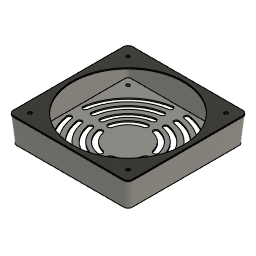
Fan Template - Tight Screen (Autodesk Fusion 360 design; units mm, degrees)
Autodesk Fusion 360 part; units mm, degrees
sketch "Base Master" plane through (0, 0, 0) normal (0, 0, 1) x (1, 0, 0)
  circle A0 centre (0, 0) radius 59.5
  line L0 (52.5, -52.5) -> (-52.5, -52.5) construction
  line L1 (-52.5, -52.5) -> (-52.5, 52.5) construction
  line L2 (-52.5, 52.5) -> (52.5, 52.5) construction
  line L3 (52.5, 52.5) -> (52.5, -52.5) construction
  line L4 (52.5, -52.5) -> (-52.5, 52.5) construction
  line L5 (-52.5, -52.5) -> (52.5, 52.5) construction
  circle A1 centre (-52.5, 52.5) radius 1.8
  circle A2 centre (52.5, 52.5) radius 1.8
  circle A3 centre (52.5, -52.5) radius 1.8
  circle A4 centre (-52.5, -52.5) radius 1.8
  line L6 (57.25, -60.25) -> (-57.25, -60.25)
  line L7 (-60.25, -57.25) -> (-60.25, 57.25)
  line L8 (-57.25, 60.25) -> (57.25, 60.25)
  line L9 (60.25, 57.25) -> (60.25, -57.25)
  line L10 (60.25, -60.25) -> (-60.25, 60.25) construction
  line L11 (-60.25, -60.25) -> (60.25, 60.25) construction
  arc A5 (-57.25, 60.25) -> (-60.25, 57.25) centre (-57.25, 57.25) ccw
  arc A6 (60.25, 57.25) -> (57.25, 60.25) centre (57.25, 57.25) ccw
  arc A7 (57.25, -60.25) -> (60.25, -57.25) centre (57.25, -57.25) ccw
  arc A8 (-60.25, -57.25) -> (-57.25, -60.25) centre (-57.25, -57.25) ccw
  line L12 (-61.85, -57.25) -> (-61.85, 57.25)
  arc A9 (-57.25, 61.85) -> (-61.85, 57.25) centre (-57.25, 57.25) ccw
  line L13 (-57.25, 61.85) -> (57.25, 61.85)
  arc A10 (61.85, 57.25) -> (57.25, 61.85) centre (57.25, 57.25) ccw
  line L14 (61.85, 57.25) -> (61.85, -57.25)
  arc A11 (57.25, -61.85) -> (61.85, -57.25) centre (57.25, -57.25) ccw
  line L15 (57.25, -61.85) -> (-57.25, -61.85)
  arc A12 (-61.85, -57.25) -> (-57.25, -61.85) centre (-57.25, -57.25) ccw
  dimension "d10" = 119
  dimension "d11" = 105
  dimension "d12" = 105
  dimension "d13" = 3.6
  dimension "d14" = 3.6
  dimension "d15" = 3.6
  dimension "d16" = 3.6
  dimension "d18" = 120.5
  dimension "d19" = 120.5
  dimension "d20" = 3
  dimension "d21" = 3
  dimension "d22" = 3
  dimension "d23" = 3
  constraint coincident A0.centre origin
  constraint horizontal L0
  constraint perpendicular L0 L1
  constraint parallel L0 L2
  constraint parallel L1 L3
  constraint coincident L4 A0.centre
  constraint coincident L5 A0.centre
  constraint coincident L1.end L2.start
  constraint coincident L2.end L3.start
  constraint coincident L0.start L3.end
  constraint coincident L0.end L1.start
  constraint horizontal L6
  constraint perpendicular L6 L7
  constraint parallel L6 L8
  constraint parallel L7 L9
  constraint coincident L10 A0.centre
  constraint coincident L11 A0.centre
  constraint coincident L10.end L7
  constraint coincident L10.end L8
  constraint tangent L7 A5
  constraint tangent L8 A5
  constraint coincident L11.end L8
  constraint coincident L11.end L9
  constraint tangent L8 A6
  constraint tangent L9 A6
  constraint coincident L10.start L9
  constraint coincident L10.start L6
  constraint tangent L9 A7
  constraint tangent L6 A7
  constraint coincident L11.start L7
  constraint coincident L11.start L6
  constraint tangent L7 A8
  constraint tangent L6 A8
  measures "d10" diameter of A0
  measures "d11" distance of L1.end L2.end
  measures "d12" distance of L0.end L1.end
  measures "d14" diameter of A1
  measures "d14" diameter of A2
  measures "d15" diameter of A4
  measures "d16" diameter of A3
  measures "d18" distance of L10.end L11.end
  measures "d19" distance of L11.start L10.end
  measures "d20" radius of A5
  measures "d21" radius of A6
  measures "d22" radius of A7
  measures "d23" radius of A8
sketch "Base Loft" plane through (0, 0, 0) normal (0, 0, 1) x (1, 0, 0)
  arc A0 (61.85, 57.25) -> (57.25, 61.85) centre (57.25, 57.25) ccw
  line L0 (61.85, 57.25) -> (61.85, -57.25)
  arc A1 (57.25, -61.85) -> (61.85, -57.25) centre (57.25, -57.25) ccw
  line L1 (57.25, -61.85) -> (-57.25, -61.85)
  arc A2 (-61.85, -57.25) -> (-57.25, -61.85) centre (-57.25, -57.25) ccw
  line L2 (-61.85, -57.25) -> (-61.85, 57.25)
  arc A3 (-57.25, 61.85) -> (-61.85, 57.25) centre (-57.25, 57.25) ccw
  line L3 (-57.25, 61.85) -> (57.25, 61.85)
  arc A4 (60.25, 57.25) -> (57.25, 60.25) centre (57.25, 57.25) ccw
  line L4 (60.25, 57.25) -> (60.25, -57.25)
  arc A5 (57.25, -60.25) -> (60.25, -57.25) centre (57.25, -57.25) ccw
  line L5 (57.25, -60.25) -> (-57.25, -60.25)
  arc A6 (-60.25, -57.25) -> (-57.25, -60.25) centre (-57.25, -57.25) ccw
  line L6 (-60.25, -57.25) -> (-60.25, 57.25)
  arc A7 (-57.25, 60.25) -> (-60.25, 57.25) centre (-57.25, 57.25) ccw
  line L7 (-57.25, 60.25) -> (57.25, 60.25)
ref_plane "WorkPlane1" through (0, 0, 26.7) normal (0, 0, 1) x (1, 0, 0)
sketch "Top Loft" plane through (0, 0, 26.7) normal (0, 0, 1) x (1, 0, 0)
  line L0 (59, -64) -> (-59, -64)
  line L1 (-64, -59) -> (-64, 59)
  line L2 (-59, 64) -> (59, 64)
  line L3 (64, 59) -> (64, -59)
  line L4 (64, -64) -> (-64, 64) construction
  line L5 (-64, -64) -> (64, 64) construction
  arc A0 (-59, 64) -> (-64, 59) centre (-59, 59) ccw
  arc A1 (64, 59) -> (59, 64) centre (59, 59) ccw
  arc A2 (-64, -59) -> (-59, -64) centre (-59, -59) ccw
  arc A3 (59, -64) -> (64, -59) centre (59, -59) ccw
  line L6 (-59, 62.4) -> (59, 62.4)
  arc A4 (62.4, 59) -> (59, 62.4) centre (59, 59) ccw
  line L7 (62.4, 59) -> (62.4, -59)
  arc A5 (59, -62.4) -> (62.4, -59) centre (59, -59) ccw
  line L8 (59, -62.4) -> (-59, -62.4)
  arc A6 (-62.4, -59) -> (-59, -62.4) centre (-59, -59) ccw
  line L9 (-62.4, -59) -> (-62.4, 59)
  arc A7 (-59, 62.4) -> (-62.4, 59) centre (-59, 59) ccw
  dimension "d27" = 128
  dimension "d28" = 128
  dimension "d29" = 5
  dimension "d30" = 5
  dimension "d31" = 5
  dimension "d32" = 5
  dimension "d33" = 1.6
  constraint horizontal L0
  constraint perpendicular L0 L1
  constraint parallel L0 L2
  constraint parallel L1 L3
  constraint coincident L4 origin
  constraint coincident L5 origin
  constraint coincident L4.end L1
  constraint coincident L4.end L2
  constraint tangent L1 A0
  constraint tangent L2 A0
  constraint coincident L5.end L2
  constraint coincident L5.end L3
  constraint tangent L2 A1
  constraint tangent L3 A1
  constraint coincident L5.start L1
  constraint coincident L5.start L0
  constraint tangent L1 A2
  constraint tangent L0 A2
  constraint coincident L4.start L3
  constraint coincident L4.start L0
  constraint tangent L3 A3
  constraint tangent L0 A3
  measures "d27" distance of L4.end L5.end
  measures "d28" distance of L5.start L4.end
  measures "d29" radius of A0
  measures "d30" radius of A1
  measures "d31" radius of A2
  measures "d32" radius of A3
loft "Loft1" add profiles "Base Loft", "Top Loft" section 1 section 2 contours L0 L1 L2 L3 A0 A1 A2 A3 | L6 A4 L7 A5 L8 A6 L9 A7 makes body 1 in component "Fan Cage"
loft "Loft2" cut profiles "Top Loft", "Base Loft" section 1 contours L6 A4 L7 A5 L8 A6 L9 A7 section 2 contours A4 L4 A5 L5 A6 L6 A7 L7 bodies 1 in component "Fan Cage"
extrude "Extrude1" add sketch "Base Master" along normal blind 1.2 contours L6 L7 L8 L9 A5 A6 A7 A8 | L12 A9 L13 A10 L14 A11 L15 A12 bodies 1 in component "Fan Cage"
sketch "Sketch4" plane through (0, 0, 0) normal (0, 0, 1) x (1, 0, 0)
  circle A0 centre (0, 0) radius 17.5
  line L0 (0, 0) -> (0, 20) construction
  line L1 (4.1758, 16.9945) -> (4.1758, 59.3533)
  line L2 (-4.1758, 16.9945) -> (-4.1758, 59.3533)
  circle A1 centre (0, 0) radius 59.5
  line L3 (-12.6298, 12.1136) -> (-49.3136, 33.293)
  line L4 (-16.8056, 4.8809) -> (-53.4893, 26.0603)
  line L5 (-16.8056, -4.8809) -> (-53.4893, -26.0603)
  line L6 (-12.6298, -12.1136) -> (-49.3136, -33.293)
  line L7 (-4.1758, -16.9945) -> (-4.1758, -59.3533)
  line L8 (4.1758, -16.9945) -> (4.1758, -59.3533)
  line L9 (12.6298, -12.1136) -> (49.3136, -33.293)
  line L10 (16.8056, -4.8809) -> (53.4893, -26.0603)
  line L11 (16.8056, 4.8809) -> (53.4893, 26.0603)
  line L12 (12.6298, 12.1136) -> (49.3136, 33.293)
  dimension "d38" = 35
  dimension "d41" = 360
  constraint coincident A0.centre L0.start
  constraint vertical L0
  constraint parallel L0 L1
  constraint coincident A0 L1.start
  constraint symmetric L0 L1.end L2.end
  constraint symmetric L0 L1.start L2.start
  constraint coincident L2.end A1
  measures "d38" diameter of A0
sketch "Sketch6" plane through (0, 0, 0) normal (0, 0, 1) x (1, 0, 0)
  circle A0 centre (0, 0) radius 59.5
  circle A1 centre (0, 0) radius 17.5
  arc A2 (21.7926, 4.8357) -> (4.8273, 21.7944) centre (0, 0) ccw
  arc A3 (21.7926, 4.8357) -> (27.0202, 5.9957) centre (24.4064, 5.4157) ccw
  arc A4 (27.0202, 5.9957) -> (5.9853, 27.0225) centre (0, 0) ccw
  arc A5 (5.9853, 27.0225) -> (4.8273, 21.7944) centre (5.4063, 24.4084) ccw
  arc A6 (24.4064, 5.4157) -> (5.4063, 24.4084) centre (0, 0) ccw construction
  line L0 (0, 0) -> (17.6743, 17.6811) construction
  line L1 (24.4064, 5.4157) -> (0, 0) construction
  line L2 (0, 0) -> (5.4063, 24.4084) construction
  arc A7 (31.5148, 5.8676) -> (5.8555, 31.517) centre (0, 0) ccw
  arc A8 (31.5148, 5.8676) -> (36.4303, 6.7828) centre (33.9725, 6.3252) ccw
  arc A9 (36.4303, 6.7828) -> (6.7688, 36.4329) centre (0, 0) ccw
  arc A10 (6.7688, 36.4329) -> (5.8555, 31.517) centre (6.3122, 33.975) ccw
  arc A11 (33.9725, 6.3252) -> (6.3122, 33.975) centre (0, 0) ccw construction
  line L3 (24.4303, 24.4397) -> (0, 0) construction
  line L4 (0, 0) -> (24.9864, 2.8019) construction
  line L5 (24.9864, 2.8019) -> (59.1294, 6.6305) construction
  line L6 (0, 0) -> (2.7923, 24.9874) construction
  line L7 (2.7923, 24.9874) -> (6.6079, 59.1319) construction
  arc A12 (7.8896, 46.8402) -> (7.0591, 41.9097) centre (7.4744, 44.3749) ccw
  arc A13 (46.8372, 7.9076) -> (7.8896, 46.8402) centre (0, 0) ccw
  arc A14 (41.9069, 7.0752) -> (46.8372, 7.9076) centre (44.3721, 7.4914) ccw
  arc A15 (41.9069, 7.0752) -> (7.0591, 41.9097) centre (0, 0) ccw
  arc A16 (44.3721, 7.4914) -> (7.4744, 44.3749) centre (0, 0) ccw construction
  line L8 (0, 0) -> (31.8137, 31.8259) construction
  arc A17 (8.9766, 56.795) -> (8.196, 51.8563) centre (8.5863, 54.3256) ccw
  arc A18 (56.7915, 8.9984) -> (8.9766, 56.795) centre (0, 0) ccw
  arc A19 (51.8531, 8.2159) -> (56.7915, 8.9984) centre (54.3223, 8.6072) ccw
  arc A20 (51.8531, 8.2159) -> (8.196, 51.8563) centre (0, 0) ccw
  arc A21 (54.3223, 8.6072) -> (8.5863, 54.3256) centre (0, 0) ccw construction
  arc A22 (-4.8357, 21.7926) -> (-21.7944, 4.8273) centre (0, 0) ccw
  arc A23 (-4.8357, 21.7926) -> (-5.9957, 27.0202) centre (-5.4157, 24.4064) ccw
  arc A24 (-5.9957, 27.0202) -> (-27.0225, 5.9853) centre (0, 0) ccw
  arc A25 (-27.0225, 5.9853) -> (-21.7944, 4.8273) centre (-24.4084, 5.4063) ccw
  arc A26 (-36.4329, 6.7688) -> (-31.517, 5.8555) centre (-33.975, 6.3122) ccw
  arc A27 (-6.7828, 36.4303) -> (-36.4329, 6.7688) centre (0, 0) ccw
  arc A28 (-5.8676, 31.5148) -> (-6.7828, 36.4303) centre (-6.3252, 33.9725) ccw
  arc A29 (-5.8676, 31.5148) -> (-31.517, 5.8555) centre (0, 0) ccw
  arc A30 (-46.8402, 7.8896) -> (-41.9097, 7.0591) centre (-44.3749, 7.4744) ccw
  arc A31 (-7.9076, 46.8372) -> (-46.8402, 7.8896) centre (0, 0) ccw
  arc A32 (-7.0752, 41.9069) -> (-7.9076, 46.8372) centre (-7.4914, 44.3721) ccw
  arc A33 (-7.0752, 41.9069) -> (-41.9097, 7.0591) centre (0, 0) ccw
  arc A34 (-56.795, 8.9766) -> (-51.8563, 8.196) centre (-54.3256, 8.5863) ccw
  arc A35 (-8.9984, 56.7915) -> (-56.795, 8.9766) centre (0, 0) ccw
  arc A36 (-8.2159, 51.8531) -> (-8.9984, 56.7915) centre (-8.6072, 54.3223) ccw
  arc A37 (-8.2159, 51.8531) -> (-51.8563, 8.196) centre (0, 0) ccw
  arc A38 (-21.7926, -4.8357) -> (-4.8273, -21.7944) centre (0, 0) ccw
  arc A39 (-21.7926, -4.8357) -> (-27.0202, -5.9957) centre (-24.4064, -5.4157) ccw
  arc A40 (-27.0202, -5.9957) -> (-5.9853, -27.0225) centre (0, 0) ccw
  arc A41 (-5.9853, -27.0225) -> (-4.8273, -21.7944) centre (-5.4063, -24.4084) ccw
  arc A42 (-6.7688, -36.4329) -> (-5.8555, -31.517) centre (-6.3122, -33.975) ccw
  arc A43 (-36.4303, -6.7828) -> (-6.7688, -36.4329) centre (0, 0) ccw
  arc A44 (-31.5148, -5.8676) -> (-36.4303, -6.7828) centre (-33.9725, -6.3252) ccw
  arc A45 (-31.5148, -5.8676) -> (-5.8555, -31.517) centre (0, 0) ccw
  arc A46 (-7.8896, -46.8402) -> (-7.0591, -41.9097) centre (-7.4744, -44.3749) ccw
  arc A47 (-46.8372, -7.9076) -> (-7.8896, -46.8402) centre (0, 0) ccw
  arc A48 (-41.9069, -7.0752) -> (-46.8372, -7.9076) centre (-44.3721, -7.4914) ccw
  arc A49 (-41.9069, -7.0752) -> (-7.0591, -41.9097) centre (0, 0) ccw
  arc A50 (-8.9766, -56.795) -> (-8.196, -51.8563) centre (-8.5863, -54.3256) ccw
  arc A51 (-56.7915, -8.9984) -> (-8.9766, -56.795) centre (0, 0) ccw
  arc A52 (-51.8531, -8.2159) -> (-56.7915, -8.9984) centre (-54.3223, -8.6072) ccw
  arc A53 (-51.8531, -8.2159) -> (-8.196, -51.8563) centre (0, 0) ccw
  arc A54 (4.8357, -21.7926) -> (21.7944, -4.8273) centre (0, 0) ccw
  arc A55 (4.8357, -21.7926) -> (5.9957, -27.0202) centre (5.4157, -24.4064) ccw
  arc A56 (5.9957, -27.0202) -> (27.0225, -5.9853) centre (0, 0) ccw
  arc A57 (27.0225, -5.9853) -> (21.7944, -4.8273) centre (24.4084, -5.4063) ccw
  arc A58 (36.4329, -6.7688) -> (31.517, -5.8555) centre (33.975, -6.3122) ccw
  arc A59 (6.7828, -36.4303) -> (36.4329, -6.7688) centre (0, 0) ccw
  arc A60 (5.8676, -31.5148) -> (6.7828, -36.4303) centre (6.3252, -33.9725) ccw
  arc A61 (5.8676, -31.5148) -> (31.517, -5.8555) centre (0, 0) ccw
  arc A62 (46.8402, -7.8896) -> (41.9097, -7.0591) centre (44.3749, -7.4744) ccw
  arc A63 (7.9076, -46.8372) -> (46.8402, -7.8896) centre (0, 0) ccw
  arc A64 (7.0752, -41.9069) -> (7.9076, -46.8372) centre (7.4914, -44.3721) ccw
  arc A65 (7.0752, -41.9069) -> (41.9097, -7.0591) centre (0, 0) ccw
  arc A66 (56.795, -8.9766) -> (51.8563, -8.196) centre (54.3256, -8.5863) ccw
  arc A67 (8.9984, -56.7915) -> (56.795, -8.9766) centre (0, 0) ccw
  arc A68 (8.2159, -51.8531) -> (8.9984, -56.7915) centre (8.6072, -54.3223) ccw
  arc A69 (8.2159, -51.8531) -> (51.8563, -8.196) centre (0, 0) ccw
  dimension "d46" = 35
  dimension "d47" = 25
  dimension "d48" = 65
  dimension "d51" = 2.5
  dimension "d53" = 2.5
  dimension "d54" = 45
  dimension "d55" = 2.5
  dimension "d57" = 55
  dimension "d59" = 360
  constraint tangent A2 A3
  constraint tangent A3 A4
  constraint tangent A4 A5
  constraint tangent A2 A5
  constraint coincident A0.centre A1.centre
  constraint midpoint A6 L0.end
  constraint coincident A3.centre A6.start
  constraint coincident A5.centre A6.end
  constraint symmetric L0 L1 L2
  constraint tangent A7 A8
  constraint tangent A8 A9
  constraint tangent A9 A10
  constraint tangent A7 A10
  constraint midpoint A11 L3.start
  constraint midpoint A3 L4.end
  constraint coincident A0 L5.end
  constraint parallel L4 L5
  constraint midpoint A5 L6.end
  constraint coincident A0 L7.end
  constraint parallel L6 L7
  constraint tangent A8 L5
  constraint tangent A14 A15
  constraint tangent A13 A14
  constraint tangent A12 A13
  constraint tangent A12 A15
  constraint midpoint A16 L8.end
  constraint tangent L5 A14
  constraint tangent A10 L7
  constraint tangent L7 A12
  constraint tangent A19 A20
  constraint tangent A18 A19
  constraint tangent A17 A18
  constraint tangent A17 A20
  constraint tangent L7 A17
  constraint tangent L5 A19
  measures "d46" diameter of A1
  measures "d47" radius of A6
  measures "d48" angle of L1 L2
  measures "d51" radius of A8
  measures "d53" radius of A14
  measures "d54" radius of A16
  measures "d55" radius of A19
  measures "d57" radius of A21
extrude "Extrude2" add sketch "Sketch6" along normal up to surface (1.2 mm away) contours A0 | A1 bodies 1 in component "Fan Cage"
sketch "Sketch5" plane through (0, 0, 26.7) normal (0, 0, 1) x (1, 0, 0)
  circle A0 centre (-52.5, 52.5) radius 1.8
  circle A1 centre (52.5, 52.5) radius 1.8
  circle A2 centre (52.5, -52.5) radius 1.8
  circle A3 centre (-52.5, -52.5) radius 1.8
  spline S0 degree 3 poles (-64, -59) (-64, -59.6532) (-63.8693, -60.3201) (-63.6081, -60.9405) (-63.2242, -61.8522) (-62.5532, -62.656) (-61.7174, -63.1971) (-60.9017, -63.7252) (-59.9368, -64) (-59, -64) (-19.6667, -64) (19.6667, -64) (59, -64) (59.6532, -64) (60.3201, -63.8693) (60.9405, -63.6081) (61.8522, -63.2242) (62.656, -62.5532) (63.1971, -61.7174) (63.7252, -60.9017) (64, -59.9368) (64, -59) (64, -19.6667) (64, 19.6667) (64, 59) (64, 59.6532) (63.8693, 60.3201) (63.6081, 60.9405) (63.2242, 61.8522) (62.5532, 62.656) (61.7174, 63.1971) (60.9017, 63.7252) (59.9368, 64) (59, 64) (19.6667, 64) (-19.6667, 64) (-59, 64) (-59.6532, 64) (-60.3201, 63.8693) (-60.9405, 63.6081) (-61.8522, 63.2242) (-62.656, 62.5532) (-63.1971, 61.7174) (-63.7252, 60.9017) (-64, 59.9368) (-64, 59) (-64, 19.6667) (-64, -19.6667) (-64, -59) knots 0 0 0 0 0.003899 0.003899 0.003899 0.009629 0.009629 0.009629 0.015221 0.015221 0.015221 0.25 0.25 0.25 0.253899 0.253899 0.253899 0.259629 0.259629 0.259629 0.265221 0.265221 0.265221 0.5 0.5 0.5 0.503899 0.503899 0.503899 0.509629 0.509629 0.509629 0.515221 0.515221 0.515221 0.75 0.75 0.75 0.753899 0.753899 0.753899 0.759629 0.759629 0.759629 0.765221 0.765221 0.765221 1 1 1 1
  circle A4 centre (0, 0) radius 59.5
extrude "Extrude1'" add sketch "Sketch5" along normal blind 1.2 separate body makes body 2 in component "TPU Gasket"
component "Fan Cage" placed x (1, 0, 0) y (0, 1, 0) z (0, 0, 1) at (0, 0, 0)
component "TPU Gasket" placed x (1, 0, 0) y (0, 1, 0) z (0, 0, 1) at (0, 0, 0)
equation "fan_dia = 120 mm" comment "Diameter of the fan itself"
equation "hole_dia = fan_dia - 1 mm" comment "Actual size of the fan hole"
equation "screw_hole_dia = 3.6 mm" comment "Screw hole size"
equation "screw_hole_spacing = 105 mm" comment "Space between screws"
equation "fillet_fan = 3 mm" comment "Radius of fan edge fillet"
equation "fillet_wide = 5 mm" comment "Radius of large edge fillet"
equation "inside_margin = 1 mm" comment "Space around fan inside cage"
equation "fan_thickness = 25 mm" comment "Thickness of fan"
equation "wide_edge = fan_dia + 8 mm" comment "Distance between widest edges"
equation "d10 = hole_dia"
equation "d11 = screw_hole_spacing"
equation "d12 = screw_hole_spacing"
equation "d13 = screw_hole_dia"
equation "d14 = d13"
equation "d15 = d13"
equation "d16 = d13"
equation "narrow_edge = fan_dia + 0.5 mm" comment "Distance between shortest edges"
equation "d18 = narrow_edge"
equation "d19 = narrow_edge"
equation "d20 = fillet_fan"
equation "d21 = fillet_fan"
equation "d22 = fillet_fan"
equation "d23 = fillet_fan"
equation "wall_thickness = 1.6 mm"
equation "d25 = -wall_thickness"
equation "d26 = fan_thickness + face_thickness + 0.5 mm"
equation "d27 = wide_edge"
equation "d28 = wide_edge"
equation "d29 = fillet_wide"
equation "d30 = fillet_wide"
equation "d31 = fillet_wide"
equation "d32 = fillet_wide"
equation "d33 = wall_thickness"
equation "face_thickness = 1.2 mm" comment "Thickness of fan face"
equation "d35 = face_thickness"
equation "motor_dia = 35 mm" comment "Area in center covered by fan motor"
equation "d38 = motor_dia"
equation "d46 = motor_dia"
